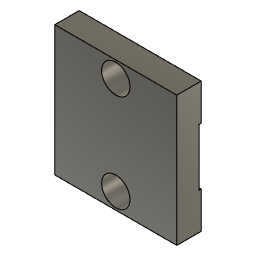
Y-Belt-Clamp (Autodesk Fusion 360 design; units mm, degrees)
Autodesk Fusion 360 part; units mm, degrees
sketch "Skizze1" plane through (0, 0, 0) normal (0, 0, 1) x (1, 0, 0)
  line L0 (0, 0) -> (15, 0)
  line L1 (15, 0) -> (15, 2)
  line L2 (1, 2) -> (0, 2)
  line L3 (0, 2) -> (0, 0)
  line L4 (13, 2) -> (13, 2.75)
  line L5 (9, 2) -> (9, 2.75)
  line L6 (5, 2) -> (5, 2.75)
  line L7 (15, 2) -> (15, 2.75)
  line L8 (1, 2) -> (2, 2)
  line L9 (2, 2) -> (3, 2)
  line L10 (3, 2) -> (4, 2)
  line L11 (4, 2) -> (5, 2)
  line L12 (5, 2) -> (6, 2)
  line L13 (6, 2) -> (7, 2)
  line L14 (7, 2) -> (8, 2)
  line L15 (8, 2) -> (9, 2)
  line L16 (9, 2) -> (10, 2)
  line L17 (10, 2) -> (11, 2)
  line L18 (11, 2) -> (12, 2)
  line L19 (12, 2) -> (13, 2)
  line L20 (13, 2) -> (14, 2)
  line L21 (14, 2) -> (15, 2)
  line L22 (15, 2.75) -> (14, 2)
  line L23 (14, 2) -> (13, 2.75)
  line L24 (13, 2.75) -> (12, 2)
  line L25 (12, 2) -> (11.0004, 2.75)
  line L26 (11.0004, 2.75) -> (10, 2)
  line L27 (10, 2) -> (9, 2.75)
  line L28 (7, 2) -> (7, 2.75)
  line L29 (3, 2) -> (3, 2.75)
  line L30 (1, 2) -> (1, 2.75)
  line L31 (9, 2.75) -> (8, 2)
  line L32 (8, 2) -> (7, 2.75)
  line L33 (7, 2.75) -> (6, 2)
  line L34 (6, 2) -> (5, 2.75)
  line L35 (5, 2.75) -> (4, 2)
  line L36 (4, 2) -> (3, 2.75)
  line L37 (3, 2.75) -> (2, 2)
  line L38 (2, 2) -> (1, 2.75)
  line L39 (1, 2.75) -> (0, 2)
  dimension "d1" = 15
  dimension "d2" = 2
  dimension "d9" = 1
  dimension "d10" = 0.75
  dimension "d11" = 0.75
  dimension "d12" = 0.75
  dimension "d13" = 0.75
  dimension "d14" = 1
  dimension "d15" = 1
  dimension "d16" = 1
  dimension "d17" = 1
  dimension "d18" = 1
  dimension "d19" = 1
  dimension "d20" = 1
  dimension "d21" = 1
  dimension "d22" = 1
  dimension "d23" = 1
  dimension "d24" = 1
  dimension "d25" = 1
  dimension "d26" = 1
  dimension "d27" = 1
  dimension "d28" = 0.75
  dimension "d29" = 0.75
  dimension "d30" = 0.75
  dimension "d31" = 0.75
  constraint coincident L0.start L3.end
  constraint horizontal L0
  constraint perpendicular L0 L1
  constraint parallel L2 L8
  constraint parallel L8 L9
  constraint parallel L9 L10
  constraint parallel L10 L11
  constraint perpendicular L6 L12
  constraint perpendicular L6 L13
  constraint parallel L13 L14
  constraint parallel L14 L15
  constraint perpendicular L5 L16
  constraint horizontal L17
  constraint parallel L17 L18
  constraint parallel L18 L19
  constraint perpendicular L4 L20
  constraint parallel L20 L21
  constraint parallel L22 L24
  constraint perpendicular L13 L28
  constraint perpendicular L9 L29
  constraint perpendicular L8 L30
  constraint parallel L33 L35
  constraint parallel L34 L36
  measures "d1" distance of L0.start L0.end
  measures "d2" distance of L1.end L4.start
  measures "d9" distance of L2.start L2.end
  measures "d10" distance of L4.start L4.end
  measures "d11" distance of L5.start L5.end
  measures "d12" distance of L6.start L6.end
  measures "d13" distance of L1.end L7.end
  measures "d14" distance of L2.start L8.end
  measures "d15" distance of L8.end L9.end
  measures "d16" distance of L9.end L10.end
  measures "d17" distance of L10.end L6.start
  measures "d18" distance of L6.start L12.end
  measures "d19" distance of L12.end L13.end
  measures "d20" distance of L13.end L14.end
  measures "d21" distance of L14.end L5.start
  measures "d22" distance of L5.start L16.end
  measures "d23" distance of L16.end L17.end
  measures "d24" distance of L17.end L18.end
  measures "d25" distance of L18.end L4.start
  measures "d26" distance of L4.start L20.end
  measures "d27" distance of L20.end L1.end
  measures "d28" distance of L17.end L25.end
  measures "d29" distance of L13.end L28.end
  measures "d30" distance of L9.end L29.end
  measures "d31" distance of L2.start L30.end
extrude "Extrusion1" add sketch "Skizze1" along normal blind 7
sketch "Skizze2" plane through (0, 0, 0) normal (0, -1, 0) x (1, 0, 0)
  line L0 (0, 0) -> (15, 0)
  line L1 (15, 0) -> (15, 7)
  line L2 (15, 7) -> (0, 7)
  line L3 (0, 7) -> (0, 0)
  line L4 (0, 7) -> (15, 7)
  line L5 (15, 7) -> (15, 11.5)
  line L6 (15, 11.5) -> (0, 11.5)
  line L7 (0, 11.5) -> (0, 7)
  line L8 (0, 0) -> (15, 0)
  line L9 (15, 0) -> (15, -4.5)
  line L10 (15, -4.5) -> (0, -4.5)
  line L11 (0, -4.5) -> (0, 0)
  line L12 (7.5, 11.5) -> (7.5, 7)
  line L13 (7.5, -4.5) -> (7.5, 0)
  circle A0 centre (7.5, 9.5) radius 1.75
  circle A1 centre (7.5, -2.5) radius 1.75
  dimension "d34" = 4.5
  dimension "d35" = 4.5
  dimension "d37" = 3.5
  dimension "d38" = 3.5
  dimension "d39" = 2.5
  dimension "d41" = 2.5
  constraint horizontal L4
  constraint vertical L5
  constraint horizontal L6
  constraint vertical L7
  constraint coincident L2.end L3.start
  constraint horizontal L8
  constraint vertical L9
  constraint horizontal L10
  constraint vertical L11
  constraint coincident L0.start L3.end
  constraint midpoint L6 L12.start
  constraint midpoint L4 L12.end
  constraint midpoint L10 L13.start
  constraint midpoint L0 L13.end
  constraint coincident L12 A0.centre
  constraint coincident L13 A1.centre
  measures "d34" distance of L2.end L6.end
  measures "d35" distance of L0.start L10.end
  measures "d37" diameter of A0
  measures "d38" diameter of A1
  measures "d39" distance of L8 A1.centre
  measures "d41" distance of L4 A0.centre
extrude "Extrusion2" add sketch "Skizze2" against normal blind 3 contours L0 L8 L10 L11 L13 A1 | L0 L8 L9 L10 L13 A1 | L2 L4 L6 L7 L12 A0 | L2 L4 L5 L6 L12 A0
